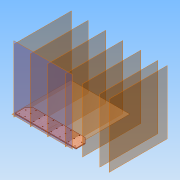
# Autodesk Inventor part: Pancake_Timing Backboard_3 Lanes
Saved by Autodesk Inventor 2018.1 (Build 221171000, 171)
## iProperties
Created: 2019-02-22
Part Number: Pancake_Timing Backboard_3 Lanes
Material: Wood (Oak)
Document SubType Name: Modeling
Designer: James
Density: 0.76 g/cm^3
Appearance: White Oak - Natural Medium Gloss
Author: James
Autodesk Inventor part; units mm, degrees
ref_plane "YZ Plane" through (0, 0, 0) normal (1, 0, 0) x (0, 1, 0)
ref_plane "XZ Plane" through (0, 0, 0) normal (0, 1, 0) x (-1, 0, 0)
ref_plane "XY Plane" through (0, 0, 0) normal (0, 0, 1) x (1, 0, 0)
derived "Pancake_Skeleton.ipt"
ref_plane "Ground" through (0, 0, 0) normal (0, 1, 0) x (-1, 0, 0)
ref_plane "Back" through (0, 0, 0) normal (0, 0, 1) x (1, 0, 0)
ref_plane "LHS" through (0, 0, 0) normal (1, 0, 0) x (0, 1, 0)
ref_plane "Lane 1" through (90, 0, 0) normal (1, 0, 0) x (0, 1, 0)
ref_plane "Lane 2" through (185, 0, 0) normal (1, 0, 0) x (0, 1, 0)
ref_plane "Lane 3" through (280, 0, 0) normal (1, 0, 0) x (0, 1, 0)
ref_plane "Lane 4" through (375, 0, 0) normal (1, 0, 0) x (0, 1, 0)
ref_plane "Lane 5" through (470, 0, 0) normal (1, 0, 0) x (0, 1, 0)
ref_plane "RHS" through (520, 0, 0) normal (1, 0, 0) x (0, 1, 0)
sketch "Sketch1" plane through (0, 0, 0) normal (0, 0, 1) x (1, 0, 0)
  line L0 (0, 60) -> (0, -10) projected
  line L1 (-66, 0) -> (396, 0) projected
  line L2 (0, 0) -> (330, 0)
  line L3 (330, 0) -> (330, 50)
  line L4 (330, 50) -> (0, 50)
  line L5 (0, 50) -> (0, 0)
  line L6 (520, 60) -> (520, -10) projected
  dimension "d1" = 50
  dimension "d30" = 190
  constraints: 8 end point, 2 parallel, 1 horizontal, 1 perpendicular
  measures "d1" distance of L2.end L3.end
  measures "d30" distance between parallel lines of L6 L3
extrude "Extrusion1" add sketch "Sketch1" along normal blind 5
sketch "Sketch2" plane through (0, 0, 5) normal (0, 0, 1) x (1, 0, 0)
  line L0 (90, 60) -> (90, -10) projected
  line L1 (330, 50) -> (0, 50) projected
  line L2 (-85, 0) -> (510, 0) projected
  line L3 (185, 60) -> (185, -10) projected
  point P0 (0, 0)
  point P1 (42.5, 40)
  point P2 (42.5, 10)
  dimension "d4" = 30
  dimension "d5" = 10
  dimension "d6" = 10
  dimension "d28" = 47.5
  dimension "d29" = 95
  constraints: 1 vertical alignment
  measures "d4" distance of point (42.5, 10) point (42.5, 40)
  measures "d5" distance from line of L1 point (42.5, 40)
  measures "d6" distance from line of L2 point (42.5, 10)
  measures "d28" distance from line of L0 point (42.5, 40)
  measures "d29" distance between parallel lines of L3 L0
hole "Hole1" at (42.5, 40, 5) at (42.5, 10, 5) direction (0, 0, -1) diameter 4.5 end through all clearance for "Socket Head Cap Screw" size "M4" standard "Ansi Metric M Profile"
pattern_linear "Rectangular Pattern1" count 6 spacing 47.5 along (1, 0, 0) of "Hole1"
sketch "Sketch3" plane through (0, 0, 5) normal (0, 0, 1) x (1, 0, 0)
  line L0 (330, 50) -> (0, 50) projected
  line L1 (-85, 0) -> (510, 0) projected
  line L2 (0, 60) -> (0, -10) projected
  point P0 (0, 0)
  point P1 (12.5, 42.5)
  point P2 (12.5, 7.5)
  dimension "d17" = 7.5
  dimension "d18" = 7.5
  dimension "d19" = 35
  dimension "d20" = 12.5
  constraints: 1 vertical alignment
  measures "d17" distance from line of L0 point (12.5, 42.5)
  measures "d18" distance from line of L1 point (12.5, 7.5)
  measures "d19" distance of point (12.5, 42.5) point (12.5, 7.5)
  measures "d20" distance from line of L2 point (12.5, 42.5)
hole "Hole2" at (12.5, 42.5, 5) at (12.5, 7.5, 5) direction (0, 0, -1) diameter 4.5 end through all clearance for "Socket Head Cap Screw" size "M4" standard "Ansi Metric M Profile"
ref_plane "Work Plane10" through (165, 0, 0) normal (-1, 0, 0) x (0, 0, 1)
mirror "Mirror1" about plane through (165, 0, 0) normal (-1, 0, 0) of "Hole2"
sketch "Sketch4" plane through (0, 0, 5) normal (0, 0, 1) x (1, 0, 0)
  line L0 (330, 50) -> (0, 50) projected
  line L1 (0, 50) -> (330, 50)
  line L2 (330, 50) -> (330, 75)
  line L3 (330, 75) -> (0, 75)
  line L4 (0, 75) -> (0, 50)
  point P0 (0, 0)
  dimension "d31" = 25
  constraints: 8 end point, 2 parallel, 1 coincident, 1 horizontal, 1 perpendicular
  measures "d31" distance of L1.end L2.end
extrude "Extrusion2" add sketch "Sketch4" against normal up to surface (5 mm away)
chamfer "Chamfer1" distance 25 angle 45 2 edges at (0, 75, 2.5) (330, 75, 2.5)
sketch "Sketch5" plane through (0, 0, 5) normal (0, 0, 1) x (1, 0, 0)
  circle A0 centre (42.5, 40) radius 2.25 projected
  line L0 (305, 75) -> (25, 75) projected
  point P0 (0, 0)
  point P1 (42.5, 69)
  dimension "d37" = 6
  constraints: 1 vertical alignment
  measures "d37" distance from line of point (42.5, 69) L0
hole "Hole3" at (42.5, 69, 5) direction (0, 0, -1) diameter 4.5 end through all clearance for "Flat Head Machine Screw" size "M4" standard "Ansi Metric M Profile"
pattern_linear "Rectangular Pattern2" count 6 spacing 47.5 along (1, 0, 0) of "Hole3"
equation "\"d5\" = d6"
equation "\"d28\" = 0.5 * d29"
equation "\"d18\" = d17"
body "Solid1"
